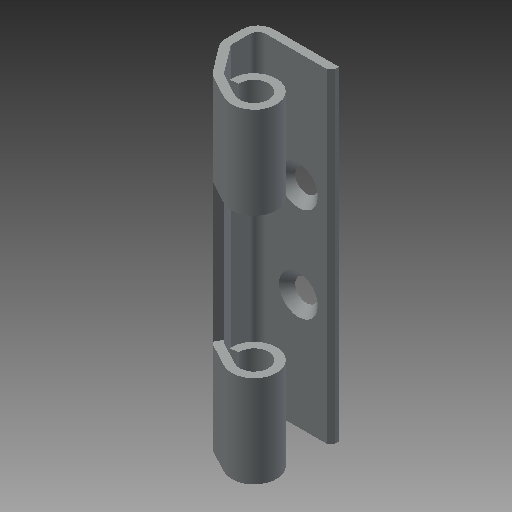
# Autodesk Inventor part: 1XXX_01_04
Saved by Autodesk Inventor 2019.3 (Build 233278000, 278)
## iProperties
Category: PARTsolutions
Company: RITTAL
Created: 2018-11-14
Part Number: 1XXX_01_04
Material: Generic
Catalog Web Link: www.cadenas.de
Description: Scharnier AE-Scharnier AE
Vendor: RITTAL
Document SubType Name: Modeling
Designer: psadmin
Manufacturer: RITTAL
Mass: 3.42976 g
Surface Area: 50.4565 cm^2
Volume: 3.42976 cm^3
Density: 1 g/cm^3
Appearance: PSOLRGB-195-201-196
PSOL_IDENT_0: {$CADENAS_DATA\23d-libs\rittal_usa\schaltschranksys\kompakt_schaltschr\ae\parts_ae\scharnier_ae.prj}
PSOL_IDENT_1: ,179 {VTYP=3D},{NB=1XXX_01_04},{LINA=1XXX_01_04},{NN=Scharnier AE},{DATE=08.11.2018 06:46:30},{GEOMD
PSOL_IDENT_2: ATE=07.07.2014 12:39:28},{VERSION=v140715130753},{LINEID=10},{WBVAR=},{WBNUMERIC=}  {NB=1XXX_01_04},
PSOL_IDENT_3: {LINA=1XXX_01_04},{KT=DUMMY},{BEST=1XXX},{VERS=1},{BEZ1=MIN},{BEZ2=MIN},{BEZ3=MIN}
NN: Scharnier AE
NT: Scharnier AE
NB: 1XXX_01_04
NBSYN: $BEST._01_04
LINA: 1XXX_01_04
BEST: 1XXX
VERS: 1
BEZ1: 0
BEZ2: 0
BEZ3: 0
SUPPLIER: RITTAL
ARTICLENO: 1XXX_01_04
BOMINFO: 1XXX_01_04
CREATOR: CADENAS GmbH
Title: 1XXX_01_04
Author: Cadenas PARTsolutions
Comments: Scharnier AE
Autodesk Inventor part; units mm, degrees
sketch "Skizze_1" plane through (0, 0, 0) normal (0, 1, 0) x (-1, 0, 0)
  arc A0 (9, 5.9981) -> (8.3959, 7.8036) centre (6, 5.9981) ccw
  line L0 (8.3959, 7.8036) -> (4.8967, 12.4471)
  arc A1 (4.8967, 12.4471) -> (3.9166, 13.2866) centre (2.5008, 10.6417) ccw
  line L1 (3.9166, 13.2866) -> (-0.1415, 15.4588)
  arc A2 (-0.1415, 15.4588) -> (2.0342, 12.1617) centre (-2.1, 11.8) ccw
  line L2 (2.0342, 12.1617) -> (0.5399, 12.031)
  arc A3 (-0.8494, 14.1363) -> (0.5399, 12.031) centre (-2.1, 11.8) ccw
  line L3 (-0.8494, 14.1363) -> (3.5, 11.8082)
  line L4 (3.5, 11.8082) -> (7.5, 6.5)
  line L5 (7.5, 6.5) -> (7.5, 3)
  arc A4 (6, 1.5) -> (7.5, 3) centre (6, 3) ccw
  line L6 (6, 1.5) -> (-5.3, 1.5)
  line L7 (-5.3, 1.5) -> (-6, 0.8)
  line L8 (-6, 0.8) -> (-6, 0)
  line L9 (-6, 0) -> (6, 0)
  arc A5 (6, 0) -> (9, 3) centre (6, 3) ccw
  line L10 (9, 3) -> (9, 5.9981)
  constraints: 22 end point, 12 point on circle, 6 centre point
extrude "Extrusion1" add sketch "Skizze_1" along normal mid plane 60
sketch "Skizze_2" plane through (0, 0, 0) normal (1, 0, 0) x (0, 1, 0)
  line L0 (8.75, 0) -> (8.75, 1.5)
  line L1 (8.75, 1.5) -> (12.35, 1.5)
  line L2 (12.35, 1.5) -> (10.85, 0)
  line L3 (10.85, 0) -> (8.75, 0)
  line L4 (8.75, 0) -> (8.75, 1.5)
  constraints: 10 end point
revolve "Revolution1" cut sketch "Skizze_2" angle 360 about axis through (0, 8.75, 0) along (0, 0, -1)
sketch "Skizze_3" plane through (0, 0, 0) normal (1, 0, 0) x (0, 1, 0)
  line L0 (-8.75, 0) -> (-8.75, 1.5)
  line L1 (-8.75, 1.5) -> (-5.15, 1.5)
  line L2 (-5.15, 1.5) -> (-6.65, 0)
  line L3 (-6.65, 0) -> (-8.75, 0)
  line L4 (-8.75, 0) -> (-8.75, 1.5)
  constraints: 10 end point
revolve "Revolution2" cut sketch "Skizze_3" angle 360 about axis through (0, -8.75, 0) along (0, 0, -1)
sketch "Skizze_5" plane through (0, 0, 0) normal (0, 1, 0) x (-1, 0, 0)
  line L0 (19.1684, 40) -> (-42.1, 40)
  line L1 (-42.1, 40) -> (-42.1, 3)
  line L2 (-42.1, 3) -> (-0.5049, 3)
  line L3 (-0.5049, 3) -> (19.1684, 40)
  constraints: 8 end point
extrude "Extrusion2" cut sketch "Skizze_5" along normal mid plane 26
ref_plane "scharnier_XY" through (0, -8.75, 0) normal (0, 0, 1) x (1, 0, 0)
ref_plane "scharnier_YZ" through (0, -8.75, 0) normal (1, 0, 0) x (0, 1, 0)
ref_plane "scharnier_ZX" through (0, -8.75, 0) normal (0, 1, 0) x (0, 0, 1)
ref_plane "scharnier_2_XY" through (0, 8.75, 0) normal (0, 0, 1) x (1, 0, 0)
ref_plane "scharnier_2_YZ" through (0, 8.75, 0) normal (1, 0, 0) x (0, 1, 0)
ref_plane "scharnier_2_ZX" through (0, 8.75, 0) normal (0, 1, 0) x (0, 0, 1)
ref_plane "tuer_XY" through (2.1, 0, 11.8) normal (0, 1, 0) x (1, 0, 0)
ref_plane "tuer_YZ" through (2.1, 0, 11.8) normal (1, 0, 0) x (0, 0, -1)
ref_plane "tuer_ZX" through (2.1, 0, 11.8) normal (0, 0, -1) x (0, 1, 0)
body "Solid1"
